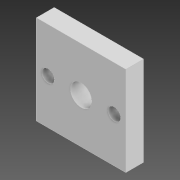
# Autodesk Inventor part: gearbox v2 top part
Saved by Autodesk Inventor 2020 (Build 240168000, 168)
## iProperties
Created: 2020-05-25
Part Number: gearbox v2 top part
Material: Generic
Document SubType Name: Modeling
Designer: stefa
Density: 1 g/cm^3
Appearance: Default
Author: stefa
Autodesk Inventor part; units mm, degrees
ref_plane "YZ Plane" through (0, 0, 0) normal (1, 0, 0) x (0, 1, 0)
ref_plane "XZ Plane" through (0, 0, 0) normal (0, 1, 0) x (-1, 0, 0)
ref_plane "XY Plane" through (0, 0, 0) normal (0, 0, 1) x (1, 0, 0)
sketch "Sketch1" plane through (0, 0, 0) normal (0, 0, 1) x (1, 0, 0)
  line L0 (-25, -25) -> (25, -25)
  line L1 (25, -25) -> (25, 25)
  line L2 (25, 25) -> (-25, 25)
  line L3 (-25, 25) -> (-25, -25)
  line L4 (-25, -25) -> (25, 25) construction
  line L5 (25, -25) -> (-25, 25) construction
  circle A0 centre (0, 0) radius 6
  circle A1 centre (18.5, 0) radius 3.5
  circle A2 centre (-18.5, 0) radius 3.5
  point P0 (25, -3.3541)
  point P1 (25, 3.3541)
  point P2 (-25, 3.3541)
  point P3 (-25, -3.3541)
  dimension "d0" = 50
  dimension "d1" = 50
  dimension "d2" = 12
  dimension "d3" = 7
  dimension "d4" = 18.5
  dimension "d5" = 18.5
  constraints: 12 end point, 4 midpoint, 3 centre point, 2 horizontal alignment, 2 parallel, 1 coincident, 1 equal radius, 1 horizontal, 1 perpendicular
  measures "d0" distance of L2.end L1.end
  measures "d1" distance of L1.end L0.end
  measures "d2" diameter of A0
  measures "d3" diameter of A1
  measures "d4" distance of A1.centre point (0, 0)
  measures "d5" distance of A2.centre point (0, 0)
extrude "Extrusion1" add sketch "Sketch1" along normal blind 10
equation "\"d5\" = d4"
body "Solid1"
